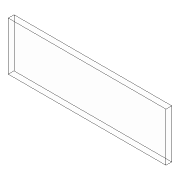
# Autodesk Inventor part: .08 Thick Polycarbonate Sheet
Saved by Autodesk Inventor 2018.3 (Build 223284000, 284)
## iProperties
Created: 2019-04-12
Part Number: .08 Thick Polycarbonate Sheet
Material: Generic
Document SubType Name: Modeling
Designer: aye06091
Mass: 1.93793 g
Surface Area: 22.0316 cm^2
Volume: 1.93793 cm^3
Density: 1 g/cm^3
Appearance: Clear - Light
Author: aye06091
Autodesk Inventor part; units mm, degrees
ref_plane "YZ Plane" through (0, 0, 0) normal (1, 0, 0) x (0, 1, 0)
ref_plane "XZ Plane" through (0, 0, 0) normal (0, 1, 0) x (-1, 0, 0)
ref_plane "XY Plane" through (0, 0, 0) normal (0, 0, 1) x (1, 0, 0)
sketch "Sketch1" plane through (0, 0, 0) normal (0, 0, 1) x (1, 0, 0)
  line L0 (0, 0) -> (55.626, 0)
  line L1 (55.626, 0) -> (55.626, -17.145)
  line L2 (55.626, -17.145) -> (0, -17.145)
  line L3 (0, -17.145) -> (0, 0)
  dimension "d0" = 55.626
  dimension "d1" = 17.145
  constraints: 8 end point, 2 parallel, 1 horizontal, 1 perpendicular
  measures "d0" distance of L0.start L0.end
  measures "d1" distance of L2.end L0.start
extrude "Extrusion1" add sketch "Sketch1" against normal blind 2.032
body "Solid1"
